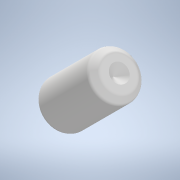
# Autodesk Inventor part: Cate2InchMecRoller
Saved by Autodesk Inventor 2020 (Build 240168000, 168)
## iProperties
Created: 2020-01-21
Part Number: Cate2InchMecRoller
Material: Generic
Document SubType Name: Modeling
Designer: srini
Density: 1 g/cm^3
Appearance: Default
Author: srini
Autodesk Inventor part; units mm, degrees
ref_plane "YZ Plane" through (0, 0, 0) normal (1, 0, 0) x (0, 1, 0)
ref_plane "XZ Plane" through (0, 0, 0) normal (0, 1, 0) x (-1, 0, 0)
ref_plane "XY Plane" through (0, 0, 0) normal (0, 0, 1) x (1, 0, 0)
sketch "Sketch2" plane through (0, 0, 0) normal (0, 0, 1) x (1, 0, 0)
  line L0 (5.1704, 7.5296) -> (-2.5593, -0.2) construction
  line L1 (0, 12.7) -> (-7.2622, 5.4378) construction
  line L2 (-7.2622, 5.4378) -> (-7.2622, 1.6155) construction
  line L3 (-5.4993, -0.2) -> (-7.2622, 1.5629) construction
  line L4 (-2.5593, -0.2) -> (-5.4993, -0.2) construction
  line L5 (0, 12.7) -> (5.1704, 7.5296) construction
  line L6 (-7.0122, 1.5957) -> (-7.0122, 5.3343)
  line L7 (-7.0122, 5.3343) -> (0.0354, 12.3818)
  line L8 (4.8875, 7.5296) -> (-2.6421, 0)
  line L9 (-2.6421, 0) -> (-5.4164, 0)
  line L10 (-5.4164, 0) -> (-7.0122, 1.5957)
  line L11 (11.1043, 19.7122) -> (7.3657, 19.7122)
  line L12 (7.3657, 19.7122) -> (0.3182, 12.6646)
  line L13 (5.1704, 7.8125) -> (12.7, 15.3421)
  line L14 (12.7, 15.3421) -> (12.7, 18.1164)
  line L15 (12.7, 18.1164) -> (11.1043, 19.7122)
  line L16 (5.1704, 7.8125) -> (4.8875, 7.5296)
  line L17 (0.3182, 12.6646) -> (0.0354, 12.3818)
  point P0 (0, 0)
  dimension "d0" = 0.25
  constraints: 26 end point, 6 symmetric about line, 1 collinear, 1 perpendicular, 1 vertical, 4 other
  measures "d0" distance between parallel lines of L1 L7
revolve "Revolution1" add sketch "Sketch2" angle 360 about axis through (7.3657, 19.7122, 0) along (-0.7071, -0.7071, 0)
fillet "Fillet1" radius 1.27 4 edges at (2.9957, 25.0464, 0) (5.77, 25.0464, 0) (-12.3464, 9.7043, 0) (-12.3464, 6.93, 0)
body "Solid1"
